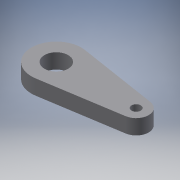
# Autodesk Inventor part: slider_link_p2
Saved by Autodesk Inventor 2017 (Build 210142000, 142)
## iProperties
Created: 2018-02-05
Part Number: slider_link_p2
Material: Generic
Document SubType Name: Modeling
Designer: Nic
Density: 1 g/cm^3
Appearance: Default
Author: Nic
Autodesk Inventor part; units mm, degrees
ref_plane "YZ Plane" through (0, 0, 0) normal (1, 0, 0) x (0, 1, 0)
ref_plane "XZ Plane" through (0, 0, 0) normal (0, 1, 0) x (-1, 0, 0)
ref_plane "XY Plane" through (0, 0, 0) normal (0, 0, 1) x (1, 0, 0)
sketch "Sketch1" plane through (0, 0, 0) normal (0, 0, 1) x (1, 0, 0)
  circle A0 centre (0, 0) radius 2.375
  line L0 (0.7812, 4.9386) -> (16.3906, 2.4693)
  arc A1 (16.3906, -2.4693) -> (16.3906, 2.4693) centre (16, 0) ccw
  line L1 (16.3906, -2.4693) -> (0.7812, -4.9386)
  arc A2 (0.7812, 4.9386) -> (0.7812, -4.9386) centre (0, 0) ccw
  circle A3 centre (16, 0) radius 0.925
  dimension "d0" = 4.75
  dimension "d3" = 2.5
  dimension "d6" = 5
  dimension "d7" = 16
  dimension "d8" = 1.85
  constraints: 5 end point, 4 centre point, 4 point on circle, 4 tangent, 2 coincident, 1 concentric, 1 horizontal alignment
  measures "d0" diameter of A0
  measures "d3" radius of A1
  measures "d6" radius of A2
  measures "d7" distance of A1.centre point (0, 0)
  measures "d8" diameter of A3
extrude "Extrusion1" add sketch "Sketch1" along normal blind 3
body "Solid1"
